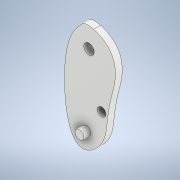
# Autodesk Inventor part: Component35
Saved by Autodesk Inventor 2022 (Build 260153000, 153)
## iProperties
Created: 2022-01-29
Part Number: Component35
Material: Generic
Document SubType Name: Modeling
Designer: Administrator
Density: 1 g/cm^3
Appearance: Default
Title: Component35
Author: Administrator
Autodesk Inventor part; units mm, degrees
ref_plane "YZ Plane" through (0, 0, 0) normal (1, 0, 0) x (0, 1, 0)
ref_plane "XZ Plane" through (0, 0, 0) normal (0, 1, 0) x (-1, 0, 0)
ref_plane "XY Plane" through (0, 0, 0) normal (0, 0, 1) x (1, 0, 0)
sketch "Sketch2" plane through (0, 0, 0) normal (0, 0, 1) x (1, 0, 0)
  circle A0 centre (1.0213, -21.0496) radius 3.175
  circle A1 centre (3.0053, 31.377) radius 3.81
  circle A2 centre (12.2184, -3.6632) radius 3.175
  spline S0 degree 5 poles (6.3065, 45.4759) (7.677, 45.1241) (10.5952, 44.1672) (15.162, 41.9307) (19.7341, 37.3848) (22.4273, 30.082) (22.3848, 22.455) (20.9622, 15.5985) (19.4596, 10.1067) (18.1899, 5.0751) (17.2105, 0.0131) (16.5389, -5.1269) (16.027, -10.2325) (15.3929, -15.1522) (14.1646, -19.9213) (11.8192, -24.6605) (8.0946, -29.1846) (3.0496, -33.0114) (-2.3177, -34.4982) (-7.0002, -32.3989) (-10.6431, -26.7916) (-13.122, -18.3209) (-14.5389, -8.09) (-15.0499, 2.6994) (-14.7475, 13.0453) (-13.6317, 22.2535) (-11.7551, 29.8998) (-9.1813, 35.7971) (-6.3126, 40.0601) (-3.3864, 42.9068) (-1.9598, 45.1095) (-0.5975, 46.235) (2.3726, 46.278) (4.9361, 45.8277) (6.3065, 45.4759) knots 0 0 0 0 0 0 0.033333 0.066667 0.1 0.133333 0.166667 0.2 0.233333 0.266667 0.3 0.333333 0.366667 0.4 0.433333 0.466667 0.5 0.533333 0.566667 0.6 0.633333 0.666667 0.7 0.733333 0.766667 0.8 0.833333 0.866667 0.9 0.933333 0.966667 1 1 1 1 1 1 weights 1 1 1 1 1 1 1 1 1 1 1 1 1 1 1 1 1 1 1 1 1 1 1 1 1 1 1 1 1 1 1 1 1 1 1
  point P0 (0, 0)
  constraints: 3 centre point, 1 other
extrude "Extrusion1" add sketch "Sketch2" along normal blind 5
sketch "Sketch3" plane through (0, 0, 5) normal (0, 0, 1) x (1, 0, 0)
  circle A0 centre (1.0213, -21.0496) radius 3.175 projected
  circle A1 centre (3.0053, 31.377) radius 3.81 projected
  circle A2 centre (12.2184, -3.6632) radius 3.175 projected
  point P0 (0, 0)
  constraints: 1 other
extrude "Extrusion2" add sketch "Sketch3" along normal blind 5 contours A0
extrude "Extrusion3" add sketch "Sketch2" along normal blind 5 contours A0
body "Solid1"
